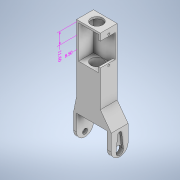
# Autodesk Inventor part: juncao2
Saved by Autodesk Inventor 2022.1 (Build 261234000, 234)
## iProperties
Created: 2021-08-02
Part Number: juncao2
Material: Generic
Document SubType Name: Modeling
Designer: nakai
Density: 1 g/cm^3
Appearance: Default
Author: nakai
Autodesk Inventor part; units mm, degrees
ref_plane "YZ Plane" through (0, 0, 0) normal (1, 0, 0) x (0, 1, 0)
ref_plane "XZ Plane" through (0, 0, 0) normal (0, 1, 0) x (-1, 0, 0)
ref_plane "XY Plane" through (0, 0, 0) normal (0, 0, 1) x (1, 0, 0)
sketch "Sketch1" plane through (0, 0, 0) normal (0, 0, 1) x (1, 0, 0)
  line L0 (0, 0) -> (24, 0)
  line L1 (24, 0) -> (24, -80)
  line L2 (24, -80) -> (0, -80)
  line L3 (0, -80) -> (0, 0)
  dimension "d0" = 24
  dimension "d1" = 80
  constraints: 8 end point, 2 parallel, 1 horizontal, 1 perpendicular
  measures "d0" distance of L1.end L2.end
  measures "d1" distance of L0.end L1.end
extrude "Extrusion1" add sketch "Sketch1" along normal blind 2
sketch "Sketch2" plane through (0, 0, 2) normal (0, 0, 1) x (1, 0, 0)
  line L0 (0, -80) -> (24, -80) projected
  line L1 (0, 0) -> (2, 0)
  line L2 (2, 0) -> (2, -80)
  line L3 (2, -80) -> (0, -80)
  line L4 (0, -80) -> (0, 0)
  line L5 (24, -80) -> (24, 0) projected
  line L6 (24, 0) -> (22, 0)
  line L7 (22, 0) -> (22, -80)
  line L8 (22, -80) -> (24, -80)
  line L9 (24, -80) -> (24, 0)
  dimension "d4" = 2
  dimension "d5" = 2
  constraints: 16 end point, 4 parallel, 2 horizontal, 2 perpendicular, 2 point on line
  measures "d4" distance of L2.end L3.end
  measures "d5" distance of L8.end L7.end
extrude "Extrusion2" add sketch "Sketch2" along normal blind 15
sketch "Sketch3" plane through (24, -80, 0) normal (1, 0, 0) x (0, 0, -1)
  circle A0 centre (-8.5, 77) radius 1
  circle A1 centre (-8.5, 49.5) radius 1
  line L0 (-17, 0) -> (-17, 80) projected
  line L1 (0, 80) -> (-17, 80) projected
  dimension "d8" = 2
  dimension "d9" = 2
  dimension "d10" = 8.5
  dimension "d11" = 8.5
  dimension "d12" = 27.5
  dimension "d13" = 3
  constraints: 2 centre point
  measures "d8" diameter of A0
  measures "d9" diameter of A1
  measures "d10" distance from line of L0 A0.centre
  measures "d11" distance from line of L0 A1.centre
  measures "d12" distance of A1.centre A0.centre
  measures "d13" distance from line of L1 A0.centre
extrude "Extrusion3" cut sketch "Sketch3" against normal up to surface (2 mm away)
sketch "Sketch4" plane through (24, -80, 0) normal (1, 0, 0) x (0, 0, -1)
  line L0 (-17, 80) -> (-17, 0) projected
  line L1 (-17, 75) -> (-2, 75)
  line L2 (-2, 75) -> (-2, 51.5)
  line L3 (-2, 51.5) -> (-17, 51.5)
  line L4 (-17, 51.5) -> (-17, 75)
  circle A0 centre (-8.5, 77) radius 1 projected
  circle A1 centre (-8.5, 49.5) radius 1 projected
  dimension "d23" = 15
  dimension "d24" = 23.5
  dimension "d25" = 2
  dimension "d26" = 2
  constraints: 8 end point, 2 parallel, 1 horizontal, 1 perpendicular, 1 point on line
  measures "d23" distance of L2.end L3.end
  measures "d24" distance of L1.end L2.end
  measures "d25" distance from line of A0.centre L1
  measures "d26" distance from line of A1.centre L3
extrude "Extrusion4" cut sketch "Sketch4" against normal up to surface (2 mm away) contours L1 L2 L3 L0
sketch "Sketch5" plane through (0, -80, 0) normal (-1, 0, 0) x (0, 0, 1)
  circle A0 centre (8.5, 68.4) radius 2.5
  circle A1 centre (8.5, 77) radius 1 projected
  point P0 (0, 80)
  dimension "d29" = 5
  dimension "d32" = 8.6
  dimension "d33" = 0
  constraints: 1 centre point
  measures "d29" diameter of A0
  measures "d32" distance of A1.centre A0.centre
  measures "d33" horizontal distance of A0.centre A1.centre
extrude "Extrusion5" add sketch "Sketch5" along normal blind 5 contours A0
sketch "Sketch12" plane through (0, 0, 0) normal (0, 0, -1) x (-1, 0, 0)
  line L0 (3, -80) -> (-35, -80)
  line L1 (-35, -80) -> (-35, -105)
  line L2 (-35, -105) -> (3, -105)
  line L3 (3, -105) -> (3, -80)
  line L4 (0, 0) -> (0, -80) projected
  line L5 (-2, -80) -> (-22, -80) projected
  line L6 (3, -80) -> (0, -80)
  line L7 (0, -80) -> (0, -105)
  line L8 (0, -105) -> (3, -105)
  line L9 (3, -105) -> (3, -80)
  line L10 (-35, -80) -> (-31, -80)
  line L11 (-31, -80) -> (-31, -105)
  line L12 (-31, -105) -> (-35, -105)
  line L13 (-35, -105) -> (-35, -80)
  dimension "d52" = 3
  dimension "d53" = 25
  dimension "d54" = 0
  dimension "d55" = 3
  dimension "d56" = 4
  dimension "d83" = 31
  constraints: 24 end point, 6 parallel, 3 horizontal, 3 perpendicular, 2 point on line
  measures "d52" distance between parallel lines of L3 L4
  measures "d53" distance between parallel lines of L2 L0
  measures "d54" distance between parallel lines of L5 L0
  measures "d55" distance of L8.end L7.end
  measures "d56" distance of L11.end L12.end
  measures "d83" distance between parallel lines of L11 L7
extrude "Extrusion9" add sketch "Sketch12" against normal up to surface (17 mm away) contours L3 L2 L7 L0 | L2 L1 L0 L11
sketch "Sketch13" plane through (0, 0, 0) normal (0, 0, -1) x (-1, 0, 0)
  line L0 (-31, -80) -> (-35, -80) projected
  line L1 (0, -80) -> (-24, -80) projected
  line L2 (-35, -80) -> (-24, -80)
  line L3 (-24, -80) -> (-24, -65)
  line L4 (-24, -65) -> (-35, -80)
  line L5 (0, -80) -> (0, -65)
  line L6 (0, 0) -> (0, -80) projected
  line L7 (0, -80) -> (15, -80) construction
  line L8 (0, -65) -> (3, -80)
  line L9 (3, -80) -> (0, -80)
  dimension "d59" = 15
  dimension "d60" = 90
  dimension "d63" = 15
  dimension "d64" = 90
  constraints: 14 end point, 3 perpendicular, 2 horizontal, 1 collinear
  measures "d59" distance of L1.end L3.end
  measures "d60" angle of L3 L2
  measures "d63" distance of L1.start L5.end
  measures "d64" angle of L7 L5
extrude "Extrusion10" add sketch "Sketch13" against normal up to surface (17 mm away)
sketch "Sketch14" plane through (-3, -105, 0) normal (-1, 0, 0) x (0, 0, 1)
  circle A0 centre (8.5, 5) radius 2.5
  line L0 (17, 0) -> (17, 25) projected
  line L1 (0, 25) -> (17, 25) projected
  point P0 (0, 105)
  dimension "d65" = 5
  dimension "d66" = 8.5
  dimension "d67" = 20
  constraints: 1 centre point
  measures "d65" diameter of A0
  measures "d66" distance from line of L0 A0.centre
  measures "d67" distance from line of L1 A0.centre
extrude "Extrusion11" cut sketch "Sketch14" against normal up to surface (38 mm away)
sketch "Sketch15" plane through (0, 0, 0) normal (0, 1, 0) x (1, 0, 0)
  line L0 (24, -17) -> (24, 0) projected
  line L1 (2, -17) -> (0, -17) projected
  line L2 (24, 0) -> (0, 0)
  line L3 (0, 0) -> (0, -17)
  line L4 (0, -17) -> (24, -17)
  line L5 (24, -17) -> (24, 0)
  constraints: 8 end point, 2 parallel, 1 horizontal, 1 perpendicular
extrude "Extrusion12" add sketch "Sketch15" along normal blind 2
sketch "Sketch16" plane through (2, -80, 2) normal (0, -1, 0) x (1, 0, 0)
  line L0 (0, 15) -> (20, 15) projected
  line L1 (0, 0) -> (20, 0) projected
  line L2 (0, 15) -> (20, 15)
  line L3 (20, 15) -> (20, 0)
  line L4 (20, 0) -> (0, 0)
  line L5 (0, 0) -> (0, 15)
  point P0 (-2, -2)
  constraints: 8 end point, 2 parallel, 1 horizontal, 1 perpendicular
extrude "Extrusion13" add sketch "Sketch16" against normal blind 46.5
sketch "Sketch17" plane through (0, 2, 0) normal (0, 1, 0) x (1, 0, 0)
  circle A0 centre (12, -8.5) radius 6
  line L0 (24, -17) -> (24, 0) projected
  line L1 (24, 0) -> (0, 0) projected
  dimension "d74" = 12
  dimension "d75" = 12
  dimension "d76" = 8.5
  constraints: 1 centre point
  measures "d74" diameter of A0
  measures "d75" distance from line of L0 A0.centre
  measures "d76" distance from line of L1 A0.centre
extrude "Extrusion14" cut sketch "Sketch17" against normal up to surface (82 mm away)
fillet "Fillet2" radius 8.5 4 edges at (33, -105, 0) (-1.5, -105, 0) (33, -105, 17) (-1.5, -105, 17)
sketch "Sketch18" plane through (35, -80, 17) normal (1, 0, 0) x (0, 0, -1)
  circle A0 centre (8.5, -20) radius 2.5 projected
  circle A1 centre (8.5, -20) radius 3.75
  point P0 (17, 80)
  dimension "d80" = 7.5
  constraints: 1 centre point, 1 coincident
  measures "d80" diameter of A1
extrude "Extrusion15" cut sketch "Sketch18" against normal up to surface (4 mm away) contours A0 | A1
sketch "Sketch20" plane through (35, -80, 17) normal (1, 0, 0) x (0, 0, -1)
  circle A0 centre (8.5, -5) radius 2
  circle A1 centre (8.5, -20) radius 3.75 projected
  line L0 (10.4863, -4.7667) -> (12.2244, -19.5625)
  line L1 (6.5137, -4.7667) -> (4.7756, -19.5625)
  circle A2 centre (8.5, -5) radius 2
  circle A3 centre (8.5, -20) radius 3.75
  line L2 (10.4863, -4.7667) -> (12.2244, -19.5625)
  line L3 (6.5137, -4.7667) -> (4.7756, -19.5625)
  point P0 (17, 80)
  dimension "d84" = 4
  dimension "d85" = 15
  dimension "d86" = 0
  dimension "d89" = 4
  dimension "d90" = 15
  dimension "d91" = 0
  constraints: 8 end point, 8 point on circle, 8 tangent, 3 centre point
  measures "d84" diameter of A0
  measures "d85" distance of A1.centre A0.centre
  measures "d86" horizontal distance of A1.centre A0.centre
  measures "d89" diameter of A2
  measures "d90" distance of A3.centre A2.centre
  measures "d91" horizontal distance of A3.centre A2.centre
extrude "Extrusion16" cut sketch "Sketch20" against normal blind 2 contours A0 | A0 L0 A1 L1
body "Solid1"
